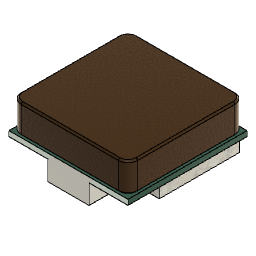
BackgroundBeacon (Autodesk Fusion 360 archive; units mm, degrees)
design "BZ-181"
Autodesk Fusion 360 part; units mm, degrees
sketch "Sketch1" plane through (0, 0, 0) normal (0, 0, 1) x (1, 0, 0)
  line L0 (-8.95, 8.95) -> (8.95, 8.95)
  line L1 (8.95, 8.95) -> (8.95, -8.95)
  line L2 (8.95, -8.95) -> (-8.95, -8.95)
  line L3 (-8.95, -8.95) -> (-8.95, 8.95)
  line L4 (-8.95, 8.95) -> (8.95, -8.95) construction
  line L5 (8.95, 8.95) -> (-8.95, -8.95) construction
  dimension "d1" = 17.9
  constraint horizontal L0
  constraint perpendicular L0 L1
  constraint parallel L0 L2
  constraint parallel L1 L3
  constraint coincident L4 origin
  constraint coincident L5 origin
  constraint equal L0 L1
  measures "d1" distance of L0.start L0.end
extrude "Extrude1" add sketch "Sketch1" against normal blind 4.5
fillet "Fillet1" radius 1.5 4 edges at (8.95, -8.95, -2.25) (-8.95, -8.95, -2.25) (-8.95, 8.95, -2.25) (8.95, 8.95, -2.25)
chamfer "Chamfer1" distance 0.25 angle 45 2 faces at (2.4833, -1.9833, 0) (2.4833, -1.9833, -4.5)
sketch "Sketch2" plane through (0, 0, -4.5) normal (0, 0, -1) x (1, 0, 0)
  arc A0 (7.45, -8.7) -> (8.7, -7.45) centre (7.45, -7.45) ccw
  line L0 (8.7, -7.45) -> (8.7, 7.45)
  arc A1 (8.7, 7.45) -> (7.45, 8.7) centre (7.45, 7.45) ccw
  line L1 (7.45, 8.7) -> (-7.45, 8.7)
  arc A2 (-7.45, 8.7) -> (-8.7, 7.45) centre (-7.45, 7.45) ccw
  line L2 (-8.7, 7.45) -> (-8.7, -7.45)
  arc A3 (-8.7, -7.45) -> (-7.45, -8.7) centre (-7.45, -7.45) ccw
  line L3 (-7.45, -8.7) -> (7.45, -8.7)
  line L4 (9.125, -9.125) -> (-9.125, -9.125)
  line L5 (-9.125, -9.125) -> (-9.125, 9.125)
  line L6 (-9.125, 9.125) -> (9.125, 9.125)
  line L7 (9.125, 9.125) -> (9.125, -9.125)
  line L8 (9.125, -9.125) -> (-9.125, 9.125) construction
  line L9 (-9.125, -9.125) -> (9.125, 9.125) construction
  dimension "d7" = 18.25
  constraint horizontal L4
  constraint perpendicular L4 L5
  constraint parallel L4 L6
  constraint parallel L5 L7
  constraint coincident L8 origin
  constraint coincident L9 origin
  constraint equal L4 L7
  measures "d7" distance of L4.start L4.end
extrude "Extrude2" add sketch "Sketch2" along normal blind 0.8 contours A0 L0 A1 L1 A2 L2 A3 L3 | L4 L5 L6 L7
sketch "Sketch3" plane through (0, 0, -5.3) normal (0, 0, -1) x (1, 0, 0)
  line L0 (9.125, 9.125) -> (-9.125, 9.125)
  line L1 (-9.125, 9.125) -> (-9.125, -9.125)
  line L2 (-9.125, -9.125) -> (9.125, -9.125)
  line L3 (9.125, -9.125) -> (9.125, 9.125)
  line L4 (-8.55, 8.55) -> (8.55, 8.55)
  line L5 (8.55, 8.55) -> (8.55, -8.55)
  line L6 (8.55, -8.55) -> (-8.55, -8.55)
  line L7 (-8.55, -8.55) -> (-8.55, 8.55)
  line L8 (-8.55, 8.55) -> (8.55, -8.55) construction
  line L9 (8.55, 8.55) -> (-8.55, -8.55) construction
  line L10 (-8.55, 3.75) -> (8.55, 3.75)
  dimension "d10" = 17.1
  dimension "d11" = 12.3
  constraint horizontal L4
  constraint perpendicular L4 L5
  constraint parallel L4 L6
  constraint parallel L5 L7
  constraint coincident L8 origin
  constraint coincident L9 origin
  constraint equal L4 L7
  constraint coincident L7 L10.start
  constraint coincident L5 L10.end
  constraint perpendicular L5 L10
  measures "d10" distance of L4.start L4.end
  measures "d11" distance of L6 L10
extrude "Extrude3" add sketch "Sketch3" along normal blind 2.1 contours L5 L6 L7 L10
sketch "Sketch4" plane through (0, 0, -5.3) normal (0, 0, -1) x (1, 0, 0)
  line L0 (-8.55, 3.75) -> (8.55, 3.75)
  line L1 (8.55, 3.75) -> (8.55, -8.55)
  line L2 (8.55, -8.55) -> (-8.55, -8.55)
  line L3 (-8.55, -8.55) -> (-8.55, 3.75)
  line L4 (9.125, 9.125) -> (-9.125, 9.125)
  line L5 (-9.125, 9.125) -> (-9.125, -9.125)
  line L6 (-9.125, -9.125) -> (9.125, -9.125)
  line L7 (9.125, -9.125) -> (9.125, 9.125)
  line L8 (3.15, 9.125) -> (-3.15, 9.125)
  line L9 (-3.15, 9.125) -> (-3.15, 4.625)
  line L10 (-3.15, 4.625) -> (3.15, 4.625)
  line L11 (3.15, 4.625) -> (3.15, 9.125)
  point P0 (0, 4.625)
  dimension "d14" = 6.3
  dimension "d15" = 4.5
  constraint horizontal L8
  constraint vertical L9
  constraint horizontal L10
  constraint vertical L11
  constraint coincident L4 L8.start
  constraint midpoint L10 P0
  constraint vertical origin P0
  measures "d14" distance of L9.end L10.end
  measures "d15" distance of L8.end L9.end
extrude "Extrude4" add sketch "Sketch4" along normal blind 3 contours L4 L8 L9 L10 L11
